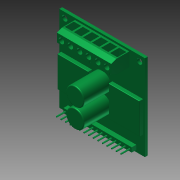
# Autodesk Inventor part: Motorcontroller
Saved by Autodesk Inventor 2012 (Build 160160000, 160)
## iProperties
Created: 2012-03-02
Part Number: Motorcontroller
Material: Default
Document SubType Name: Modeling
Designer: Lauszus
Density: 1 g/cm^3
Author: Lauszus
Autodesk Inventor part; units mm, degrees
ref_plane "YZ Plane" through (0, 0, 0) normal (1, 0, 0) x (0, 1, 0)
ref_plane "XZ Plane" through (0, 0, 0) normal (0, 1, 0) x (-1, 0, 0)
ref_plane "XY Plane" through (0, 0, 0) normal (0, 0, 1) x (1, 0, 0)
sketch "Sketch1" plane through (0, 0, 0) normal (0, 0, 1) x (1, 0, 0)
  line L0 (-25.6886, 41.0165) -> (21.5554, 41.0165)
  line L1 (21.5554, 41.0165) -> (21.5554, -6.2275)
  line L2 (21.5554, -6.2275) -> (-25.6886, -6.2275)
  line L3 (-25.6886, -6.2275) -> (-25.6886, 41.0165)
  circle A0 centre (-22.6886, 38.0165) radius 1.5
  circle A1 centre (18.5554, 38.0165) radius 1.5
  line L4 (12.9321, 32.5165) -> (-17.0679, 32.5165)
  line L5 (-17.0679, 32.5165) -> (-17.0679, 40.0165)
  line L6 (-17.0679, 40.0165) -> (12.9321, 40.0165)
  line L7 (12.9321, 40.0165) -> (12.9321, 32.5165)
  line L8 (-7.0679, 32.5165) -> (-7.0679, 40.0165)
  line L9 (2.9321, 40.0165) -> (2.9321, 32.5165)
  line L10 (-7.6886, 4.0165) -> (-24.6886, 4.0165)
  line L11 (-24.6886, 4.0165) -> (-24.6886, 21.0165)
  line L12 (-24.6886, 21.0165) -> (-7.6886, 21.0165)
  line L13 (-7.6886, 21.0165) -> (-7.6886, 4.0165)
  line L14 (3.5554, 21.0165) -> (20.5554, 21.0165)
  line L15 (20.5554, 21.0165) -> (20.5554, 4.0165)
  line L16 (20.5554, 4.0165) -> (3.5554, 4.0165)
  line L17 (3.5554, 4.0165) -> (3.5554, 21.0165)
  line L18 (-20.9134, -5.1978) -> (16.7866, -5.1978)
  line L19 (16.7866, -5.1978) -> (16.7866, -2.6978)
  line L20 (16.7866, -2.6978) -> (-20.9134, -2.6978)
  line L21 (-20.9134, -2.6978) -> (-20.9134, -5.1978)
  line L22 (15.4611, -3.6945) -> (15.9611, -3.6945)
  line L23 (15.9611, -3.6945) -> (15.9611, -4.1945)
  line L24 (15.9611, -4.1945) -> (15.4611, -4.1945)
  line L25 (15.4611, -4.1945) -> (15.4611, -3.6945)
  line L26 (12.9211, -3.6945) -> (13.4211, -3.6945)
  line L27 (13.4211, -3.6945) -> (13.4211, -4.1945)
  line L28 (13.4211, -4.1945) -> (12.9211, -4.1945)
  line L29 (12.9211, -4.1945) -> (12.9211, -3.6945)
  line L30 (7.8411, -3.6945) -> (8.3411, -3.6945)
  line L31 (8.3411, -3.6945) -> (8.3411, -4.1945)
  line L32 (8.3411, -4.1945) -> (7.8411, -4.1945)
  line L33 (7.8411, -4.1945) -> (7.8411, -3.6945)
  line L34 (10.3811, -3.6945) -> (10.8811, -3.6945)
  line L35 (10.8811, -3.6945) -> (10.8811, -4.1945)
  line L36 (10.8811, -4.1945) -> (10.3811, -4.1945)
  line L37 (10.3811, -4.1945) -> (10.3811, -3.6945)
  line L38 (5.3011, -3.6945) -> (5.8011, -3.6945)
  line L39 (5.8011, -3.6945) -> (5.8011, -4.1945)
  line L40 (5.8011, -4.1945) -> (5.3011, -4.1945)
  line L41 (5.3011, -4.1945) -> (5.3011, -3.6945)
  line L42 (2.7611, -3.6945) -> (3.2611, -3.6945)
  line L43 (3.2611, -3.6945) -> (3.2611, -4.1945)
  line L44 (3.2611, -4.1945) -> (2.7611, -4.1945)
  line L45 (2.7611, -4.1945) -> (2.7611, -3.6945)
  line L46 (0.2211, -3.6945) -> (0.7211, -3.6945)
  line L47 (0.7211, -3.6945) -> (0.7211, -4.1945)
  line L48 (0.7211, -4.1945) -> (0.2211, -4.1945)
  line L49 (0.2211, -4.1945) -> (0.2211, -3.6945)
  line L50 (-2.3189, -3.6945) -> (-1.8189, -3.6945)
  line L51 (-1.8189, -3.6945) -> (-1.8189, -4.1945)
  line L52 (-1.8189, -4.1945) -> (-2.3189, -4.1945)
  line L53 (-2.3189, -4.1945) -> (-2.3189, -3.6945)
  line L54 (-4.8589, -3.6945) -> (-4.3589, -3.6945)
  line L55 (-4.3589, -3.6945) -> (-4.3589, -4.1945)
  line L56 (-4.3589, -4.1945) -> (-4.8589, -4.1945)
  line L57 (-4.8589, -4.1945) -> (-4.8589, -3.6945)
  line L58 (-7.3989, -3.6945) -> (-6.8989, -3.6945)
  line L59 (-6.8989, -3.6945) -> (-6.8989, -4.1945)
  line L60 (-6.8989, -4.1945) -> (-7.3989, -4.1945)
  line L61 (-7.3989, -4.1945) -> (-7.3989, -3.6945)
  line L62 (-9.9389, -3.6945) -> (-9.4389, -3.6945)
  line L63 (-9.4389, -3.6945) -> (-9.4389, -4.1945)
  line L64 (-9.4389, -4.1945) -> (-9.9389, -4.1945)
  line L65 (-9.9389, -4.1945) -> (-9.9389, -3.6945)
  line L66 (-12.4789, -3.6945) -> (-11.9789, -3.6945)
  line L67 (-11.9789, -3.6945) -> (-11.9789, -4.1945)
  line L68 (-11.9789, -4.1945) -> (-12.4789, -4.1945)
  line L69 (-12.4789, -4.1945) -> (-12.4789, -3.6945)
  line L70 (-15.0189, -3.6945) -> (-14.5189, -3.6945)
  line L71 (-14.5189, -3.6945) -> (-14.5189, -4.1945)
  line L72 (-14.5189, -4.1945) -> (-15.0189, -4.1945)
  line L73 (-15.0189, -4.1945) -> (-15.0189, -3.6945)
  line L74 (-17.5589, -3.6945) -> (-17.0589, -3.6945)
  line L75 (-17.0589, -3.6945) -> (-17.0589, -4.1945)
  line L76 (-17.0589, -4.1945) -> (-17.5589, -4.1945)
  line L77 (-17.5589, -4.1945) -> (-17.5589, -3.6945)
  line L78 (-20.097, -3.6945) -> (-19.597, -3.6945)
  line L79 (-19.597, -3.6945) -> (-19.597, -4.1945)
  line L80 (-19.597, -4.1945) -> (-20.097, -4.1945)
  line L81 (-20.097, -4.1945) -> (-20.097, -3.6945)
  circle A2 centre (-2.0689, 7.6933) radius 5
  circle A3 centre (-2.0689, 18.3228) radius 5
  circle A4 centre (-14.5265, 36.2665) radius 1.5
  circle A5 centre (-9.6093, 36.2665) radius 1.5
  circle A6 centre (0.3907, 36.2665) radius 1.5
  circle A7 centre (-4.5265, 36.2665) radius 1.5
  circle A8 centre (5.4735, 36.2665) radius 1.5
  circle A9 centre (10.3907, 36.2665) radius 1.5
  line L82 (-6.6886, 25.5165) -> (-12.6886, 25.5165)
  line L83 (-12.6886, 25.5165) -> (-12.6886, 31.5165)
  line L84 (-12.6886, 31.5165) -> (-6.6886, 31.5165)
  line L85 (-6.6886, 31.5165) -> (-6.6886, 25.5165)
  line L86 (4.5554, 25.5165) -> (-1.4446, 25.5165)
  line L87 (-1.4446, 25.5165) -> (-1.4446, 31.5165)
  line L88 (-1.4446, 31.5165) -> (4.5554, 31.5165)
  line L89 (4.5554, 31.5165) -> (4.5554, 25.5165)
  point P0 (0, 0)
  dimension "d0" = 47.244
  dimension "d1" = 47.244
  dimension "d2" = 3
  dimension "d3" = 3
  dimension "d4" = 3
  dimension "d5" = 3
  dimension "d6" = 3
  dimension "d7" = 3
  dimension "d8" = 30
  dimension "d9" = 10
  dimension "d10" = 10
  dimension "d11" = 8.6208
  dimension "d12" = 1
  dimension "d13" = 7.5
  dimension "d14" = 37.7
  dimension "d15" = 4.7752
  dimension "d16" = 17
  dimension "d17" = 17
  dimension "d18" = 17
  dimension "d19" = 17
  dimension "d20" = 20
  dimension "d21" = 20
  dimension "d23" = 0.5
  dimension "d24" = 0.5
  dimension "d25" = 0.5
  dimension "d26" = 0.5
  dimension "d27" = 0.5
  dimension "d28" = 0.5
  dimension "d29" = 0.5
  dimension "d30" = 0.5
  dimension "d31" = 0.5
  dimension "d32" = 0.5
  dimension "d33" = 0.5
  dimension "d34" = 0.5
  dimension "d35" = 0.5
  dimension "d36" = 0.5
  dimension "d37" = 0.5
  dimension "d38" = 0.5
  dimension "d39" = 0.5
  dimension "d40" = 0.5
  dimension "d41" = 0.5
  dimension "d42" = 0.5
  dimension "d43" = 0.5
  dimension "d44" = 0.5
  dimension "d45" = 0.5
  dimension "d46" = 0.5
  dimension "d47" = 0.5
  dimension "d48" = 0.5
  dimension "d49" = 0.5
  dimension "d50" = 0.5
  dimension "d51" = 0.5
  dimension "d52" = 0.5
  dimension "d53" = 0.8255
  dimension "d54" = 2.54
  dimension "d55" = 2.54
  dimension "d56" = 2.54
  dimension "d57" = 2.54
  dimension "d58" = 2.54
  dimension "d59" = 2.54
  dimension "d60" = 2.54
  dimension "d61" = 2.54
  dimension "d62" = 2.54
  dimension "d63" = 2.54
  dimension "d64" = 2.54
  constraints: 180 end point, 44 parallel, 24 perpendicular, 22 horizontal, 10 centre point, 4 point on line
  measures "d0" distance of L2.end L0.start
  measures "d1" distance of L1.end L2.end
  measures "d2" diameter of A0
  measures "d3" diameter of A1
  measures "d4" distance from line of L3 A0.centre
  measures "d5" distance from line of L0 A0.centre
  measures "d6" distance from line of L1 A1.centre
  measures "d7" distance from line of L0 A1.centre
  measures "d8" distance between parallel lines of L7 L5
  measures "d9" distance between parallel lines of L7 L9
  measures "d10" distance between parallel lines of L8 L9
  measures "d11" distance between parallel lines of L3 L5
  measures "d12" distance between parallel lines of L0 L6
  measures "d13" distance between parallel lines of L6 L4
  measures "d14" distance of L18.start L18.end
  measures "d15" distance between parallel lines of L3 L21
  measures "d16" distance of L14.end L15.end
  measures "d17" distance of L12.end L10.start
  measures "d18" distance of L14.start L14.end
  measures "d19" distance of L11.end L12.end
  measures "d20" distance between parallel lines of L0 L12
  measures "d21" distance between parallel lines of L0 L14
  measures "d23" distance of L22.start L22.end
  measures "d24" distance of L22.end L23.end
  measures "d25" distance of L29.end L27.start
  measures "d26" distance of L27.start L27.end
  measures "d27" distance of L33.end L31.start
  measures "d28" distance of L31.start L31.end
  measures "d29" distance of L37.end L35.start
  measures "d30" distance of L35.start L35.end
  measures "d31" distance of L41.end L39.start
  measures "d32" distance of L39.start L39.end
  measures "d33" distance of L45.end L43.start
  measures "d34" distance of L43.start L43.end
  measures "d35" distance of L49.end L47.start
  measures "d36" distance of L47.start L47.end
  measures "d37" distance of L53.end L51.start
  measures "d38" distance of L51.start L51.end
  measures "d39" distance of L57.end L55.start
  measures "d40" distance of L55.start L55.end
  measures "d41" distance of L61.end L59.start
  measures "d42" distance of L59.start L59.end
  measures "d43" distance of L65.end L63.start
  measures "d44" distance of L63.start L63.end
  measures "d45" distance of L69.end L67.start
  measures "d46" distance of L67.start L67.end
  measures "d47" distance of L73.end L71.start
  measures "d48" distance of L71.start L71.end
  measures "d49" distance of L77.end L75.start
  measures "d50" distance of L75.start L75.end
  measures "d51" distance of L81.end L79.start
  measures "d52" distance of L79.start L79.end
  measures "d53" distance from line of L19 L22.end
  measures "d54" distance between parallel lines of L27 L23
  measures "d55" distance between parallel lines of L35 L27
  measures "d56" distance between parallel lines of L31 L35
  measures "d57" distance between parallel lines of L39 L31
  measures "d58" distance between parallel lines of L43 L39
  measures "d59" distance between parallel lines of L47 L43
  measures "d60" distance between parallel lines of L51 L47
  measures "d61" distance between parallel lines of L55 L51
  measures "d62" distance between parallel lines of L59 L55
  measures "d63" distance between parallel lines of L63 L59
  measures "d64" distance between parallel lines of L67 L63
extrude "Extrusion1" add sketch "Sketch1" along normal blind 2.5 contours L21 L20 L19 L18
extrude "Extrusion2" add sketch "Sketch1" along normal blind 7.5 contours L22 L23 L24 L25 | L26 L27 L28 L29 | L30 L31 L32 L33 | L34 L35 L36 L37 | L38 L39 L40 L41 | L42 L43 L44 L45 | L46 L47 L48 L49 | L50 L51 L52 L53 | L54 L55 L56 L57 | L58 L59 L60 L61 | L62 L63 L64 L65 | L66 L67 L68 L69 | L70 L71 L72 L73 | L74 L75 L76 L77 | L78 L79 L80 L81
extrude "Extrusion3" add sketch "Sketch1" along normal blind 2 contours L10 L11 L12 L13 | L14 L15 L16 L17
extrude "Extrusion4" add sketch "Sketch1" along normal blind 10 contours L4 L9 L6 L7 | L4 L8 L6 L9 | L4 L5 L6 L8
extrude "Extrusion5" add sketch "Sketch1" along normal blind 7.5 contours A4 | A5 | A6 | A7 | A8 | A9
extrude "Extrusion6" add sketch "Sketch1" along normal blind 15 contours A2 | A3
fillet "Fillet1" radius 0.508 2 edges at (-7.0689, 18.3228, 15) (-7.0689, 7.6933, 15)
fillet "Fillet2" radius 0.254 8 edges at (-24.6886, 12.5165, 2) (-16.1886, 4.0165, 2) (-7.6886, 12.5165, 2) (-16.1886, 21.0165, 2) (20.5554, 12.5165, 2) (12.0554, 21.0165, 2) (3.5554, 12.5165, 2) (12.0554, 4.0165, 2)
chamfer "Chamfer1" distance 1.778 angle 60 1 edges at (-2.0679, 32.5165, 10) measured on face at (-2.0679, 33.0165, 10)
chamfer "Chamfer2" distance 1.016 angle 70 1 edges at (-2.0679, 40.0165, 10) measured on face at (-2.0679, 39.5165, 10)
sketch "Sketch2" plane through (-17.0679, 40.0165, 0) normal (0, 1, 0) x (1, 0, 0)
  line L0 (30, 0) -> (0, 0) projected
  line L1 (0, 0) -> (0, -7.2086) projected
  line L2 (25.5, -1.1049) -> (29.5, -1.1049)
  line L3 (29.5, -1.1049) -> (29.5, -6.1049)
  line L4 (29.5, -6.1049) -> (25.5, -6.1049)
  line L5 (25.5, -6.1049) -> (25.5, -1.1049)
  line L6 (24.5, -6.1049) -> (20.5, -6.1049)
  line L7 (20.5, -6.1049) -> (20.5, -1.1049)
  line L8 (20.5, -1.1049) -> (24.5, -1.1049)
  line L9 (24.5, -1.1049) -> (24.5, -6.1049)
  line L10 (19.5, -6.1049) -> (15.5, -6.1049)
  line L11 (15.5, -6.1049) -> (15.5, -1.1049)
  line L12 (15.5, -1.1049) -> (19.5, -1.1049)
  line L13 (19.5, -1.1049) -> (19.5, -6.1049)
  line L14 (14.5, -6.1049) -> (10.5, -6.1049)
  line L15 (10.5, -6.1049) -> (10.5, -1.1049)
  line L16 (10.5, -1.1049) -> (14.5, -1.1049)
  line L17 (14.5, -1.1049) -> (14.5, -6.1049)
  line L18 (9.5, -6.1049) -> (5.5, -6.1049)
  line L19 (5.5, -6.1049) -> (5.5, -1.1049)
  line L20 (5.5, -1.1049) -> (9.5, -1.1049)
  line L21 (9.5, -1.1049) -> (9.5, -6.1049)
  line L22 (4.5, -6.1049) -> (0.5, -6.1049)
  line L23 (0.5, -6.1049) -> (0.5, -1.1049)
  line L24 (0.5, -1.1049) -> (4.5, -1.1049)
  line L25 (4.5, -1.1049) -> (4.5, -6.1049)
  point P0 (17.0679, 0)
  dimension "d121" = 1
  dimension "d122" = 1
  dimension "d123" = 1
  dimension "d124" = 1
  dimension "d125" = 1
  dimension "d126" = 4
  dimension "d127" = 4
  dimension "d128" = 4
  dimension "d129" = 4
  dimension "d130" = 4
  dimension "d131" = 4
  dimension "d132" = 5
  dimension "d133" = 5
  dimension "d134" = 5
  dimension "d135" = 5
  dimension "d136" = 5
  dimension "d137" = 5
  dimension "d138" = 1.1049
  dimension "d139" = 1.1049
  dimension "d140" = 1.1049
  dimension "d141" = 1.1049
  dimension "d142" = 1.1049
  dimension "d143" = 1.1049
  dimension "d144" = 0.5
  constraints: 48 end point, 12 parallel, 6 horizontal, 6 perpendicular
  measures "d121" distance between parallel lines of L19 L25
  measures "d122" distance between parallel lines of L15 L21
  measures "d123" distance between parallel lines of L11 L17
  measures "d124" distance between parallel lines of L7 L13
  measures "d125" distance between parallel lines of L5 L9
  measures "d126" distance of L3.end L4.end
  measures "d127" distance of L6.start L6.end
  measures "d128" distance of L10.start L10.end
  measures "d129" distance of L14.start L14.end
  measures "d130" distance of L18.start L18.end
  measures "d131" distance of L22.start L22.end
  measures "d132" distance between parallel lines of L4 L2
  measures "d133" distance of L8.end L6.start
  measures "d134" distance of L22.end L23.end
  measures "d135" distance of L18.end L19.end
  measures "d136" distance of L14.end L15.end
  measures "d137" distance of L12.end L10.start
  measures "d138" distance between parallel lines of L0 L24
  measures "d139" distance between parallel lines of L0 L12
  measures "d140" distance between parallel lines of L0 L8
  measures "d141" distance between parallel lines of L0 L20
  measures "d142" distance between parallel lines of L0 L16
  measures "d143" distance between parallel lines of L0 L2
  measures "d144" distance between parallel lines of L1 L23
extrude "Extrusion7" cut sketch "Sketch2" against normal blind 6
extrude "Extrusion8" add sketch "Sketch1" against normal blind 1.6 contours L0 L1 L2 L3 | L4 L9 L6 L7 | L4 L8 L6 L9 | L4 L5 L6 L8 | L10 L11 L12 L13 | L14 L15 L16 L17 | L21 L20 L19 L18 | L22 L23 L24 L25 | L26 L27 L28 L29 | L30 L31 L32 L33 | L34 L35 L36 L37 | L38 L39 L40 L41 | L42 L43 L44 L45 | L46 L47 L48 L49 | L50 L51 L52 L53 | L54 L55 L56 L57 | L58 L59 L60 L61 | L62 L63 L64 L65 | L66 L67 L68 L69 | L70 L71 L72 L73 | L74 L75 L76 L77 | L78 L79 L80 L81 | A2 | A3 | A4 | A5 | A6 | A7 | A8 | A9 | L82 L83 L84 L85 | L86 L87 L88 L89
extrude "Extrusion9" add sketch "Sketch1" along normal blind 2.5 contours L82 L83 L84 L85 | L86 L87 L88 L89
fillet "Fillet3" radius 0.254 8 edges at (-6.6886, 28.5165, 2.5) (-9.6886, 31.5165, 2.5) (-12.6886, 28.5165, 2.5) (-9.6886, 25.5165, 2.5) (1.5554, 25.5165, 2.5) (-1.4446, 28.5165, 2.5) (1.5554, 31.5165, 2.5) (4.5554, 28.5165, 2.5)
body "Solid1"
